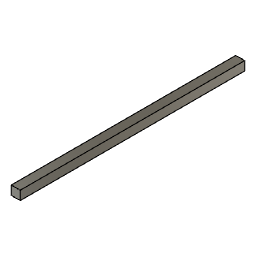
ADR Taskphase build version 1 v1 (Autodesk Fusion 360 archive; units mm, degrees)
design "arms2"
Autodesk Fusion 360 part; units mm, degrees
sketch "Sketch1" plane through (0, 0, 0) normal (0, 1, 0) x (1, 0, 0)
  line L0 (5, -5) -> (-5, -5)
  line L1 (-5, -5) -> (-5, 5)
  line L2 (-5, 5) -> (5, 5)
  line L3 (5, 5) -> (5, -5)
  line L4 (5, -5) -> (-5, 5) construction
  dimension "d1" = 10
  dimension "d2" = 10
  constraint horizontal L0
  constraint perpendicular L0 L1
  constraint parallel L0 L2
  constraint parallel L1 L3
  constraint coincident L4 origin
  measures "d1" distance of L1.end L2.end
  measures "d2" distance of L0.end L1.end
extrude "Extrude1" add sketch "Sketch1" along normal blind 250

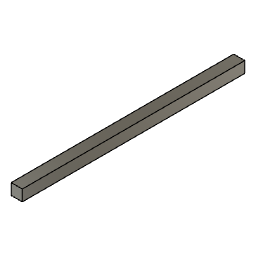
design "gear2"
Autodesk Fusion 360 part; units mm, degrees
sketch "Sketch1" plane through (0, 0, 0) normal (0, 1, 0) x (1, 0, 0)
  line L0 (5, -5) -> (-5, -5)
  line L1 (-5, -5) -> (-5, 5)
  line L2 (-5, 5) -> (5, 5)
  line L3 (5, 5) -> (5, -5)
  line L4 (5, -5) -> (-5, 5) construction
  line L5 (-5, -5) -> (5, 5) construction
  dimension "d1" = 10
  dimension "d2" = 10
  constraint horizontal L0
  constraint perpendicular L0 L1
  constraint parallel L0 L2
  constraint parallel L1 L3
  constraint coincident L4 origin
  constraint coincident L5 origin
  measures "d1" distance of L1.end L2.end
  measures "d2" distance of L0.end L1.end
extrude "Extrude1" add sketch "Sketch1" along normal blind 200

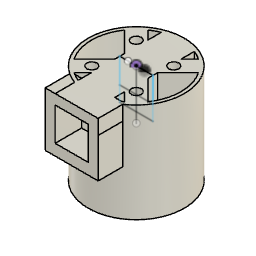
design "motor mount"
Autodesk Fusion 360 part; units mm, degrees
sketch "Sketch1" plane through (0, 0, 0) normal (0, 0, 1) x (1, 0, 0)
  circle A0 centre (0, 0) radius 8
  circle A1 centre (0, 0) radius 9.5
  line L0 (0, 0) -> (5.6569, 5.6569)
  line L1 (0, 0) -> (8, 0) construction
  line L2 (0, 0) -> (5.6569, -5.6569)
  line L3 (0, 0) -> (8.3207, 0) construction
  circle A2 centre (5.6569, 5.6569) radius 1.5
  line L4 (5.6569, -5.6569) -> (6.7175, -6.7175)
  line L5 (5.6569, -5.6569) -> (8.9706, -5.6569) construction
  circle A3 centre (6.7175, -6.7175) radius 1.5
  line L6 (0, 0) -> (-6.7175, 6.7175)
  line L7 (0, 0) -> (10.596, 0) construction
  circle A4 centre (-6.7175, 6.7175) radius 1.5
  line L8 (0, 0) -> (-6.7175, -6.7175)
  line L9 (0, 0) -> (10.7484, 0) construction
  circle A5 centre (-6.7175, -6.7175) radius 1.5
  line L10 (0, 0) -> (1.7678, 1.7678)
  line L11 (0, 0) -> (-1.7678, -1.7678)
  line L12 (-1.7678, -1.7678) -> (-8.2485, 4.713)
  line L13 (-1.7678, -1.7678) -> (7.6131, -11.1486)
  circle A6 centre (0, 0) radius 13.5
  line L14 (-8.2485, 4.713) -> (-11.1486, 7.6131)
  line L15 (1.7678, 1.7678) -> (1.4057, 2.1299)
  line L16 (1.4057, 2.1299) -> (-7.6131, 11.1486)
  line L17 (1.7678, 1.7678) -> (11.1486, -7.6131)
  line L18 (0, 0) -> (-1.7678, 1.7678)
  line L19 (-1.7678, 1.7678) -> (7.6131, 11.1486)
  line L20 (-1.7678, 1.7678) -> (-11.1486, -7.6131)
  line L21 (0, 0) -> (1.7678, -1.7678)
  line L22 (1.7678, -1.7678) -> (11.1486, 7.6131)
  line L23 (1.7678, -1.7678) -> (-7.6131, -11.1486)
  circle A7 centre (0, 0) radius 14.5
  line L24 (0, 0) -> (0, -14.5)
  dimension "d1" = 16
  dimension "d2" = 19
  dimension "d3" = 45
  dimension "d4" = 45
  dimension "d5" = 3
  dimension "d6" = 45
  dimension "d7" = 3
  dimension "d8" = 135
  dimension "d9" = 3
  dimension "d10" = 135
  dimension "d11" = 3
  dimension "d12" = 2.5
  dimension "d13" = 2.5
  dimension "d14" = 27
  dimension "d15" = 2.5
  dimension "d16" = 2.5
  dimension "d17" = 29
  constraint coincident A0.centre A1.centre
  constraint concentric A0 A1
  constraint horizontal L1
  constraint coincident A0 L0.end
  constraint horizontal L3
  constraint coincident A0 L2.end
  constraint coincident L0.end A2.centre
  constraint horizontal L5
  constraint coincident A1 L4.end
  constraint coincident L4.end A3.centre
  constraint horizontal L7
  constraint coincident A1 L6.end
  constraint coincident L6.end A4.centre
  constraint horizontal L9
  constraint coincident A1 L8.end
  constraint coincident L8.end A5.centre
  constraint parallel L0 L10
  constraint perpendicular L6 L11
  constraint coincident A1 L12.end
  constraint perpendicular L8 L12
  constraint perpendicular L11 L13
  constraint concentric A0 A6
  constraint coincident A6 L14.end
  constraint parallel L12 L14
  constraint perpendicular L0 L15
  constraint coincident A6 L16.end
  constraint perpendicular L0 L16
  constraint coincident A6 L17.end
  constraint perpendicular L0 L17
  constraint coincident A6 L13.end
  constraint perpendicular L11 L18
  constraint coincident A6 L19.end
  constraint perpendicular L6 L19
  constraint coincident A6 L20.end
  constraint perpendicular L6 L20
  constraint perpendicular L0 L21
  constraint coincident A6 L22.end
  constraint perpendicular L21 L22
  constraint coincident A6 L23.end
  constraint perpendicular L21 L23
  constraint coincident A7 L24.end
  constraint vertical L24
  measures "d1" diameter of A0
  measures "d2" diameter of A1
  measures "d3" angle of L0 L1
  measures "d4" angle of L2 L3
  measures "d5" diameter of A2
  measures "d6" angle of L4 L5
  measures "d7" diameter of A3
  measures "d8" angle of L6 L7
  measures "d9" diameter of A4
  measures "d10" angle of L8 L9
  measures "d11" diameter of A5
  measures "d12" distance of A0.centre L10.end
  measures "d13" distance of A0.centre L11.end
  measures "d14" diameter of A6
  measures "d15" distance of A0.centre L18.end
  measures "d16" distance of A0.centre L21.end
  measures "d17" diameter of A7
extrude "Extrude1" add sketch "Sketch1" against normal blind 30 contours A0 L0 A2 L17 L22 | A0 A1 A2 L22 | A0 A1 A3 L17 | A0 L2 L17 L22 | L0 L2 L10 L17 L21 L22 | A1 A6 L19 L22 | A0 A1 A3 L13 | A0 L2 L13 L23 | A1 A3 L13 A6 L17 | A0 L0 A2 L15 L16 L19 | L0 L6 L10 L15 L16 L18 L19 | L2 L21 L23 L24 | A0 A1 A2 L19 | L6 L8 L11 L12 L18 L20 | L8 L11 L13 L24 | A0 L8 L13 L23 | A0 L6 L12 L20 | A0 L6 L16 L19 | A0 L8 L12 L20 | A0 A1 A5 L23 | A0 A1 A4 L16 | A1 A4 A6 L14 L16 | A0 A1 A4 L12 | A0 A1 A5 L20 | A1 A5 A6 L20 L23 | A7 makes body 1
sketch "Sketch2" plane through (0, 0, 0) normal (0, 1, 0) x (1, 0, 0)
  line L0 (0, 0) -> (0, 15)
  line L1 (0, 0) -> (2.5, 0)
  line L2 (-2.5, 0) -> (0, 0)
  line L3 (0, 0) -> (5, 0)
  line L4 (5, 0) -> (5, 7.5)
  line L5 (5, 7.5) -> (-5, 7.5)
  line L6 (-5, 7.5) -> (-5, 0)
  line L7 (-5, 0) -> (0, 0)
  line L8 (-5, 0) -> (-5, 12)
  line L9 (-5, 12) -> (5, 12)
  line L10 (5, 12) -> (5, 0)
  dimension "d20" = 2.5
  dimension "d23" = 7.5
  dimension "d24" = 10
  dimension "d33" = 12
  constraint coincident L0.start L1.start
  constraint vertical L0
  constraint perpendicular L0 L1
  constraint perpendicular L0 L2
  constraint perpendicular L0 L3
  constraint perpendicular L3 L4
  constraint perpendicular L0 L5
  constraint perpendicular L3 L6
  constraint perpendicular L6 L7
  constraint perpendicular L7 L8
  constraint perpendicular L0 L9
  constraint perpendicular L3 L10
  measures "d20" distance of L0.start L1.end
  measures "d23" distance of L3.end L4.end
  measures "d24" distance of L4.end L5.end
  measures "d33" distance of L6.end L8.end
extrude "Extrude2" add sketch "Sketch2" against normal blind 19.5 contours L0 L2 L5 L6 L7 L8 | L0 L1 L3 L4 L5 L10 bodies 1
extrude "Extrude3" add sketch "Sketch2" along normal blind 13.5 contours L0 L2 L5 L6 L7 L8 | L0 L1 L3 L4 L5 L10 bodies 1
sketch "Sketch3" plane through (0, -19.5, 0) normal (0, -1, 0) x (1, 0, 0)
  line L0 (5, 0) -> (-5, 0)
  line L1 (-5, 0) -> (-5, -7.5)
  line L2 (-5, -7.5) -> (5, -7.5)
  line L3 (5, -7.5) -> (5, 0)
  line L4 (-5, 0) -> (-5, -0.8052)
  line L5 (0, 0) -> (0, -3)
  line L6 (0, -3) -> (5, -3)
  line L7 (0, -3) -> (-5, -3)
  line L8 (-5, -3) -> (-5, -13)
  line L9 (-5, -13) -> (5, -13)
  line L10 (5, -13) -> (5, -3)
  line L11 (5, -4.437) -> (8, -4.437)
  line L12 (8, -4.437) -> (8, 0)
  line L13 (8, 0) -> (-5, 0)
  line L14 (-5, 0) -> (-8, 0)
  line L15 (-8, 0) -> (-8, -16.3484)
  line L16 (0, -13) -> (0, -13.3484)
  line L17 (0, -13.3484) -> (0, -16.3484)
  line L18 (0, -16.3484) -> (-8, -16.3484)
  line L19 (0, -16.3484) -> (8, -16.3484)
  line L20 (8, -4.437) -> (8, -16.3484)
  dimension "d41" = 3
  dimension "d42" = 5
  dimension "d43" = 10
  dimension "d44" = 3
  dimension "d45" = 3
  dimension "d46" = 3
  constraint coincident L1 L4.end
  constraint coincident L5.start origin
  constraint perpendicular L0 L5
  constraint perpendicular L5 L6
  constraint coincident L1 L7.end
  constraint perpendicular L1 L7
  constraint perpendicular L2 L8
  constraint perpendicular L8 L9
  constraint coincident L10 L11.start
  constraint perpendicular L10 L11
  constraint perpendicular L11 L12
  constraint parallel L0 L13
  constraint coincident L0.end L1.start
  constraint perpendicular L4 L14
  constraint perpendicular L14 L15
  constraint midpoint L9 L16.start
  constraint perpendicular L9 L16
  constraint perpendicular L9 L17
  constraint perpendicular L15 L18
  constraint perpendicular L17 L19
  constraint perpendicular L19 L20
  measures "d41" distance of L5.start L5.end
  measures "d42" distance of L5.end L6.end
  measures "d43" distance of L7.end L8.end
  measures "d44" distance of L11.start L11.end
  measures "d45" distance of L0.end L14.end
  measures "d46" distance of L16.end L17.end
extrude "Extrude6" add sketch "Sketch3" against normal blind 8 bodies 1
extrude "Extrude7" cut sketch "Sketch3" against normal blind 10 contours L1 L2 L3 L6 L7 L8 L10 | L2 L8 L9 L10 bodies 1
extrude "Extrude8" cut 1 faces at (-1.6667, -9.5, -4.5) along direction (0, 1, 0) blind 7 on bodies 1 bodies 1
sketch "Sketch4" plane through (0, 0, -30) normal (0, 0, -1) x (1, 0, 0)
  line L0 (-3.5355, 0) -> (-11.1486, -7.6131)
  arc A0 (-11.1486, 7.6131) -> (-11.1486, -7.6131) centre (0, 0) ccw
  line L1 (-11.1486, 7.6131) -> (-3.5355, 0)
  circle A1 centre (5.6569, -5.6569) radius 1.5
  arc A2 (-7.6131, -11.1486) -> (7.6131, -11.1486) centre (0, 0) ccw
  line L2 (-7.6131, -11.1486) -> (0, -3.5355)
  line L3 (0, -3.5355) -> (7.6131, -11.1486)
  circle A3 centre (-6.7175, 6.7175) radius 1.5
  circle A4 centre (-6.7175, -6.7175) radius 1.5
  line L4 (3.5355, 0) -> (11.1486, 7.6131)
  arc A5 (11.1486, -7.6131) -> (11.1486, 7.6131) centre (0, 0) ccw
  line L5 (11.1486, -7.6131) -> (3.5355, 0)
  circle A6 centre (6.7175, 6.7175) radius 1.5
  arc A7 (7.6131, 11.1486) -> (-7.6131, 11.1486) centre (0, 0) ccw
  line L6 (7.6131, 11.1486) -> (0, 3.5355)
  line L7 (0, 3.5355) -> (-7.6131, 11.1486)
  circle A8 centre (0, 0) radius 14.5
  circle A9 centre (0, 0) radius 13.5
  line L8 (-11.1486, 7.6131) -> (7.6131, -11.1486)
  line L9 (-7.6131, -11.1486) -> (-7.1464, -10.6819)
  line L10 (11.1486, 7.6131) -> (-7.6131, -11.1486)
  line L11 (7.6131, 11.1486) -> (-11.1486, -7.6131)
  line L12 (-7.6131, 11.1486) -> (11.1486, -7.6131)
  dimension "d53" = 27
  constraint concentric A0 A9
  constraint coincident A0.start L1.start
  constraint coincident A2.end L3.end
  constraint coincident A2.start L2.start
  constraint coincident L2 L9.end
  constraint perpendicular L8 L9
  constraint coincident L4.end A5.end
  constraint coincident A7.start L6.start
  constraint coincident L0.end A0.end
  constraint coincident A7.end L7.end
  constraint coincident A5.start L5.start
  measures "d53" diameter of A9
extrude "Extrude9" cut sketch "Sketch4" against normal blind 10 contours L0 L2 A9 L8 L9 L10 L11 | L1 L7 A9 L8 L11 L12 | L3 L5 A9 L8 L10 L12 | L4 L6 A9 L10 L11 L12 bodies 1
extrude "Extrude10" cut 1 faces at (0, -1.1785, -30) along direction (0, 0, 1) blind 10 on bodies 1 bodies 1
sketch "Sketch5" plane through (0, 0, 0) normal (0, 0, 1) x (-1, 0, 0)
  arc A0 (7.6131, 11.1486) -> (7.0711, 11.5) centre (0, 0) ccw
  line L0 (7.6131, 11.1486) -> (5, 8.5355)
  line L1 (5, 8.5355) -> (5, 11.5)
  line L2 (5, 11.5) -> (5, 12.5399)
  arc A1 (7.0711, 11.5) -> (5, 12.5399) centre (0, 0) ccw
  arc A2 (8, 12.0934) -> (5, 13.6107) centre (0, 0) ccw
  line L3 (5, 13.6107) -> (5, 19.5)
  line L4 (5, 19.5) -> (-8, 19.5)
  line L5 (-8, 19.5) -> (-8, 12.0934)
  arc A3 (-8, 12.0934) -> (8, 12.0934) centre (0, 0) ccw
  line L6 (-5, -4.3083) -> (-5, -7.0054)
  arc A4 (-5, -4.3083) -> (-5, -7.0054) centre (-5.6569, -5.6569) ccw
  line L7 (-7.0711, 11.5) -> (-5, 11.5)
  line L8 (-5, 11.5) -> (-5, 8.5355)
  line L9 (-5, 8.5355) -> (-7.6131, 11.1486)
  arc A5 (-7.0711, 11.5) -> (-7.6131, 11.1486) centre (0, 0) ccw
  circle A6 centre (6.7175, 6.7175) radius 1.5
  circle A7 centre (6.7175, -6.7175) radius 1.5
  circle A8 centre (-6.7175, 6.7175) radius 1.5
  line L10 (-5, -1.4645) -> (-11.1486, -7.6131)
  arc A9 (-11.1486, 7.6131) -> (-11.1486, -7.6131) centre (0, 0) ccw
  line L11 (-11.1486, 7.6131) -> (-5, 1.4645)
  line L12 (-5, 1.4645) -> (-5, -1.4645)
  line L13 (5, -12.5399) -> (5, -8.5355)
  line L14 (5, -8.5355) -> (7.6131, -11.1486)
  arc A10 (5, -12.5399) -> (7.6131, -11.1486) centre (0, 0) ccw
  line L15 (5, -1.4645) -> (5, 1.4645)
  line L16 (5, 1.4645) -> (11.1486, 7.6131)
  arc A11 (11.1486, -7.6131) -> (11.1486, 7.6131) centre (0, 0) ccw
  line L17 (11.1486, -7.6131) -> (5, -1.4645)
  arc A12 (-7.6131, -11.1486) -> (-5, -12.5399) centre (0, 0) ccw
  line L18 (-7.6131, -11.1486) -> (-5, -8.5355)
  line L19 (-5, -8.5355) -> (-5, -12.5399)
  line L20 (-5, -1.4645) -> (-3.5355, 0)
  line L21 (-5, 1.4645) -> (-3.5355, 0)
  line L22 (-5, 1.4645) -> (-5, -1.4645)
  line L23 (5, 1.4645) -> (5, -1.4645)
  line L24 (3.5355, 0) -> (3.6807, -0.1451)
  line L25 (3.6807, -0.1451) -> (5, -1.4645)
  line L26 (5, 1.4645) -> (3.5355, 0)
  line L27 (0.0007, -3.5348) -> (3.6081, -7.1423)
  line L28 (3.6081, -7.1423) -> (-3.6067, -7.1423)
  line L29 (-3.6067, -7.1423) -> (0.0007, -3.5348)
  line L30 (0.0007, 3.5298) -> (3.6081, 7.1372)
  line L31 (3.6081, 7.1372) -> (-3.6067, 7.1372)
  line L32 (-3.6067, 7.1372) -> (0.0007, 3.5298)
  circle A13 centre (0, 0) radius 8
  line L33 (3.6807, -0.1451) -> (3.5355, 0)
  dimension "d58" = 16
  constraint coincident L10.start L12.end
  constraint parallel L10 L20
  constraint coincident L11.end L12.start
  constraint perpendicular L20 L21
  constraint coincident L15.end L16.start
  constraint coincident L15.start L17.end
  constraint perpendicular L16 L25
  constraint perpendicular L25 L26
  constraint perpendicular L26 L27
  constraint horizontal L28
  constraint perpendicular L27 L29
  constraint perpendicular L27 L30
  constraint parallel L28 L31
  constraint perpendicular L30 L32
  constraint coincident A0.centre A1.centre
  constraint perpendicular L26 L33
  measures "d58" diameter of A13
copy_body "Body->Comp1" bodies 1 removing the originals makes body 2 in component "motor mount"
sketch "Sketch6" plane through (0, 0, 0) normal (0, 0, 1) x (-1, 0, 0)
  arc A0 (7.6131, 11.1486) -> (7.0711, 11.5) centre (0, 0) ccw
  line L0 (7.6131, 11.1486) -> (5, 8.5355)
  line L1 (5, 8.5355) -> (5, 11.5)
  line L2 (5, 11.5) -> (5, 12.5399)
  arc A1 (7.0711, 11.5) -> (5, 12.5399) centre (0, 0) ccw
  arc A2 (8, 12.0934) -> (5, 13.6107) centre (0, 0) ccw
  line L3 (5, 13.6107) -> (5, 19.5)
  line L4 (5, 19.5) -> (-8, 19.5)
  line L5 (-8, 19.5) -> (-8, 12.0934)
  arc A3 (-8, 12.0934) -> (8, 12.0934) centre (0, 0) ccw
  line L6 (-5, -4.3083) -> (-5, -7.0054)
  arc A4 (-5, -4.3083) -> (-5, -7.0054) centre (-5.6569, -5.6569) ccw
  line L7 (-7.0711, 11.5) -> (-5, 11.5)
  line L8 (-5, 11.5) -> (-5, 8.5355)
  line L9 (-5, 8.5355) -> (-7.6131, 11.1486)
  arc A5 (-7.0711, 11.5) -> (-7.6131, 11.1486) centre (0, 0) ccw
  circle A6 centre (6.7175, 6.7175) radius 1.5
  circle A7 centre (6.7175, -6.7175) radius 1.5
  circle A8 centre (-6.7175, 6.7175) radius 1.5
  line L10 (-5, -1.4645) -> (-11.1486, -7.6131)
  arc A9 (-11.1486, 7.6131) -> (-11.1486, -7.6131) centre (0, 0) ccw
  line L11 (-11.1486, 7.6131) -> (-5, 1.4645)
  line L12 (-5, 1.4645) -> (-5, -1.4645)
  line L13 (5, -12.5399) -> (5, -8.5355)
  line L14 (5, -8.5355) -> (7.6131, -11.1486)
  arc A10 (5, -12.5399) -> (7.6131, -11.1486) centre (0, 0) ccw
  line L15 (5, -1.4645) -> (5, 1.4645)
  line L16 (5, 1.4645) -> (11.1486, 7.6131)
  arc A11 (11.1486, -7.6131) -> (11.1486, 7.6131) centre (0, 0) ccw
  line L17 (11.1486, -7.6131) -> (5, -1.4645)
  arc A12 (-7.6131, -11.1486) -> (-5, -12.5399) centre (0, 0) ccw
  line L18 (-7.6131, -11.1486) -> (-5, -8.5355)
  line L19 (-5, -8.5355) -> (-5, -12.5399)
  circle A13 centre (-5.6569, -5.6569) radius 1.5102
  line L20 (-5, -7.0054) -> (-5, -4.3083)
  constraint concentric A4 A13
  constraint coincident L6.end A4.end
  constraint coincident L6.start A4.start
extrude "Extrude1'" cut sketch "Sketch6" against normal blind 42 contours A13 bodies 2 in component "motor mount"
component "motor mount" placed x (1, 0, 0) y (0, 1, 0) z (0, 0, 1) at (0, 0, 0)

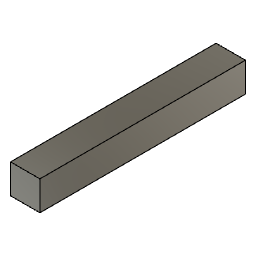
design "landing gear"
Autodesk Fusion 360 part; units mm, degrees
sketch "Sketch1" plane through (0, 0, 0) normal (0, 1, 0) x (1, 0, 0)
  line L0 (5, -5) -> (-5, -5)
  line L1 (-5, -5) -> (-5, 5)
  line L2 (-5, 5) -> (5, 5)
  line L3 (5, 5) -> (5, -5)
  line L4 (5, -5) -> (-5, 5) construction
  line L5 (-5, -5) -> (5, 5) construction
  dimension "d1" = 10
  dimension "d2" = 10
  constraint horizontal L0
  constraint perpendicular L0 L1
  constraint parallel L0 L2
  constraint parallel L1 L3
  constraint coincident L4 origin
  constraint coincident L5 origin
  measures "d1" distance of L1.end L2.end
  measures "d2" distance of L0.end L1.end
extrude "Extrude1" add sketch "Sketch1" along normal blind 70

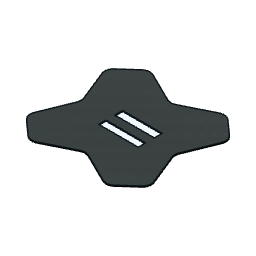
design "baseplate bse medini"
Autodesk Fusion 360 part; units mm, degrees
sketch "Sketch1" plane through (0, 0, 2) normal (0, 0, 1) x (-1, 0, 0)
  line L0 (134.7615, -76.9991) -> (106.995, -8.0888)
  line L1 (39.161, -27.8208) -> (-50, -27.8208)
  line L2 (-50, -27.8208) -> (-50, -10)
  line L3 (-50, -10) -> (39.161, -10)
  line L4 (39.161, -10) -> (39.161, -27.8208)
  line L5 (39.161, 9.6205) -> (-50, 9.6205)
  line L6 (-50, 9.6205) -> (-50, 26.3)
  line L7 (-50, 26.3) -> (39.161, 26.3)
  line L8 (39.161, 26.3) -> (39.161, 9.6205)
  line L9 (-60, -40) -> (-81.5591, -40)
  line L10 (-81.5591, -40) -> (-81.5591, 49.3306)
  line L11 (-81.5591, 49.3306) -> (-60, 49.3306)
  line L12 (-60, 49.3306) -> (-60, -40)
  line L13 (60, -40) -> (81.5591, -40)
  line L14 (60, 49.3306) -> (60, -40)
  line L15 (81.5591, -40) -> (81.5591, 49.3306)
  line L16 (81.5591, 49.3306) -> (60, 49.3306)
  line L17 (129.567, -99.3605) -> (97.0681, -128.5184)
  line L18 (74.8519, -131.5623) -> (8.8599, -98.9538)
  line L19 (-74.8519, -131.5623) -> (-8.8599, -98.9538)
  line L20 (-129.567, -99.3605) -> (-97.0681, -128.5184)
  line L21 (-134.7615, -76.9991) -> (-106.995, -8.0888)
  line L22 (129.567, 98.1323) -> (97.0681, 127.2903)
  line L23 (134.7615, 75.771) -> (106.995, 6.8607)
  line L24 (74.8519, 130.3341) -> (8.8599, 97.7257)
  line L25 (-74.8519, 130.3341) -> (-8.8599, 97.7257)
  line L26 (-134.7615, 75.771) -> (-106.995, 6.8607)
  line L27 (-129.567, 98.1323) -> (-97.0681, 127.2903)
  arc A0 (74.8519, -131.5623) -> (97.0681, -128.5184) centre (83.7118, -113.6318) ccw
  arc A1 (129.567, -99.3605) -> (134.7615, -76.9991) centre (116.2108, -84.4738) ccw
  arc A2 (8.8599, -98.9538) -> (-8.8599, -98.9538) centre (0, -116.8843) ccw
  arc A3 (-97.0681, -128.5184) -> (-74.8519, -131.5623) centre (-83.7118, -113.6318) ccw
  arc A4 (-134.7615, -76.9991) -> (-129.567, -99.3605) centre (-116.2108, -84.4738) ccw
  arc A5 (-129.567, 98.1323) -> (-134.7615, 75.771) centre (-116.2108, 83.2457) ccw
  arc A6 (-74.8519, 130.3341) -> (-97.0681, 127.2903) centre (-83.7118, 112.4036) ccw
  arc A7 (97.0681, 127.2903) -> (74.8519, 130.3341) centre (83.7118, 112.4036) ccw
  arc A8 (134.7615, 75.771) -> (129.567, 98.1323) centre (116.2108, 83.2457) ccw
  arc A9 (106.995, 6.8607) -> (106.995, -8.0888) centre (125.5457, -0.6141) ccw
  arc A10 (-106.995, -8.0888) -> (-106.995, 6.8607) centre (-125.5457, -0.6141) ccw
  arc A11 (-8.8599, 97.7257) -> (8.8599, 97.7257) centre (0, 115.6561) ccw
  arc A12 (8.8599, -98.9538) -> (-8.8599, -98.9538) centre (0, -116.8843) ccw
  arc A13 (50, 26.3) -> (46.3, 30) centre (46.3, 26.3) ccw
  line L28 (50, 26.3) -> (50, -27.8208)
  arc A14 (46.3, -31.5208) -> (50, -27.8208) centre (46.3, -27.8208) ccw
  line L29 (46.3, -31.5208) -> (39.161, -31.5208)
  arc A15 (35.461, -27.8208) -> (39.161, -31.5208) centre (39.161, -27.8208) ccw
  line L30 (35.461, -27.8208) -> (35.461, 26.3)
  arc A16 (39.161, 30) -> (35.461, 26.3) centre (39.161, 26.3) ccw
  line L31 (39.161, 30) -> (46.3, 30)
  arc A17 (24.836, 26.5208) -> (29.836, 31.5208) centre (24.836, 31.5208) ccw
  line L32 (24.836, 26.5208) -> (-25, 26.5208)
  arc A18 (-30, 31.5208) -> (-25, 26.5208) centre (-25, 31.5208) ccw
  line L33 (-30, 31.5208) -> (-30, 35)
  arc A19 (-25, 40) -> (-30, 35) centre (-25, 35) ccw
  line L34 (-25, 40) -> (24.836, 40)
  arc A20 (29.836, 35) -> (24.836, 40) centre (24.836, 35) ccw
  line L35 (29.836, 35) -> (29.836, 31.5208)
  arc A21 (-39.161, -31.5208) -> (-35.461, -27.8208) centre (-39.161, -27.8208) ccw
  line L36 (-39.161, -31.5208) -> (-46.3, -31.5208)
  arc A22 (-50, -27.8208) -> (-46.3, -31.5208) centre (-46.3, -27.8208) ccw
  line L37 (-50, -27.8208) -> (-50, 26.3)
  arc A23 (-46.3, 30) -> (-50, 26.3) centre (-46.3, 26.3) ccw
  line L38 (-46.3, 30) -> (-39.161, 30)
  arc A24 (-35.461, 26.3) -> (-39.161, 30) centre (-39.161, 26.3) ccw
  line L39 (-35.461, 26.3) -> (-35.461, -27.8208)
  line L40 (-30, -35) -> (-30, -31.5208)
  arc A25 (-25, -26.5208) -> (-30, -31.5208) centre (-25, -31.5208) ccw
  line L41 (-25, -26.5208) -> (24.836, -26.5208)
  arc A26 (29.836, -31.5208) -> (24.836, -26.5208) centre (24.836, -31.5208) ccw
  line L42 (29.836, -31.5208) -> (29.836, -35)
  arc A27 (24.836, -40) -> (29.836, -35) centre (24.836, -35) ccw
  line L43 (24.836, -40) -> (-25, -40)
  arc A28 (-30, -35) -> (-25, -40) centre (-25, -35) ccw
  line L44 (3.1623, -61.0541) -> (64.5684, -81.5228)
  arc A29 (64.5684, -81.5228) -> (69.6851, -80.3149) centre (66.1495, -76.7794) ccw
  line L45 (69.6851, -80.3149) -> (90.5258, -59.4742)
  arc A30 (90.5258, -59.4742) -> (91.6327, -54.0817) centre (86.9903, -55.9386) ccw
  line L46 (91.6327, -54.0817) -> (71.4856, -3.7139)
  arc A31 (71.4856, 3.7139) -> (71.4856, -3.7139) centre (80.7703, 0) ccw
  line L47 (71.4856, 3.7139) -> (91.6327, 54.0817)
  arc A32 (91.6327, 54.0817) -> (90.5258, 59.4742) centre (86.9903, 55.9386) ccw
  line L48 (90.5258, 59.4742) -> (69.6851, 80.3149)
  arc A33 (69.6851, 80.3149) -> (64.5684, 81.5228) centre (66.1495, 76.7794) ccw
  line L49 (64.5684, 81.5228) -> (3.1623, 61.0541)
  arc A34 (-3.1623, 61.0541) -> (3.1623, 61.0541) centre (0, 70.5409) ccw
  line L50 (-3.1623, 61.0541) -> (-64.5684, 81.5228)
  arc A35 (-64.5684, 81.5228) -> (-69.6851, 80.3149) centre (-66.1495, 76.7794) ccw
  line L51 (-69.6851, 80.3149) -> (-90.5258, 59.4742)
  arc A36 (-90.5258, 59.4742) -> (-91.6327, 54.0817) centre (-86.9903, 55.9386) ccw
  line L52 (-91.6327, 54.0817) -> (-71.4856, 3.7139)
  arc A37 (-71.4856, -3.7139) -> (-71.4856, 3.7139) centre (-80.7703, 0) ccw
  line L53 (-71.4856, -3.7139) -> (-91.6327, -54.0817)
  arc A38 (-91.6327, -54.0817) -> (-90.5258, -59.4742) centre (-86.9903, -55.9386) ccw
  line L54 (-90.5258, -59.4742) -> (-69.6851, -80.3149)
  arc A39 (-69.6851, -80.3149) -> (-64.5684, -81.5228) centre (-66.1495, -76.7794) ccw
  line L55 (-64.5684, -81.5228) -> (-3.1623, -61.0541)
  arc A40 (3.1623, -61.0541) -> (-3.1623, -61.0541) centre (0, -70.5409) ccw
  dimension "d1" = 20
  dimension "d2" = 20
  dimension "d3" = 20
  dimension "d4" = 20
  constraint horizontal L1
  constraint vertical L2
  constraint horizontal L3
  constraint vertical L4
  constraint horizontal L5
  constraint vertical L6
  constraint horizontal L7
  constraint vertical L8
  constraint horizontal L9
  constraint vertical L10
  constraint horizontal L11
  constraint vertical L12
  constraint tangent L17 A0
  constraint tangent L18 A0
  constraint tangent L0 A1
  constraint tangent L17 A1
  constraint equal A0 A1
  constraint tangent L19 A2
  constraint tangent L18 A2
  constraint equal A0 A2
  constraint tangent L19 A3
  constraint tangent L20 A3
  constraint equal A0 A3
  constraint tangent L20 A4
  constraint tangent L21 A4
  constraint equal A0 A4
  constraint tangent L26 A5
  constraint tangent L27 A5
  constraint equal A0 A5
  constraint tangent L25 A6
  constraint tangent L27 A6
  constraint equal A0 A6
  constraint tangent L22 A7
  constraint tangent L24 A7
  constraint equal A0 A7
  constraint tangent L22 A8
  constraint tangent L23 A8
  constraint equal A0 A8
  constraint tangent L0 A9
  constraint tangent L23 A9
  constraint tangent L21 A10
  constraint tangent L26 A10
  constraint tangent L24 A11
  constraint tangent L25 A11
  constraint coincident L18 A2.start
  constraint coincident L19 A2.end
  constraint tangent L18 A12
  constraint tangent L19 A12
  constraint equal A11 A12
  measures "d1" radius of A0
  measures "d2" radius of A9
  measures "d3" radius of A10
  measures "d4" radius of A11
extrude "Extrude1" add sketch "Sketch1" along normal blind 2 contours L0 L17 L18 L19 L20 L21 L22 L23 L24 L25 L26 L27 A0 A1 A2 A3 A4 A5 A6 A7 A8 A9 A10 A11 A12 | L1 L3 L4 L5 L7 L8 A13 L28 A14 L29 A15 L30 A16 L31 | L1 L40 A25 A26 L42 A27 L43 A28 | L3 L5 L30 L39 | L3 L5 L37 L39 | L1 A21 L36 A22 | L7 A23 L38 A24 | L9 L10 L11 L12 L13 L14 L15 L16 L44 A29 L45 A30 L46 L47 A32 L48 A33 L49 A34 L50 A35 L51 A36 L52 L53 A38 L54 A39 L55 A40 | L9 L10 L11 L12 L52 A37 L53 | L10 L52 A37 L53 | L15 L46 A31 L47 | L13 L14 L15 L16 L46 A31 L47 | A17 L32 A18 L33 A19 L34 A20 L35
sketch "Sketch2" plane through (0, 0, 0) normal (1, 0, 0) x (0, 1, 0)
sketch "Sketch3" plane through (0, 0, 4) normal (0, 0, 1) x (-1, 0, 0)
  line L0 (39.161, -27.8208) -> (-50, -27.8208)
  line L1 (-50, -27.8208) -> (-50, -10)
  line L2 (-50, -10) -> (39.161, -10)
  line L3 (39.161, -10) -> (39.161, -27.8208)
  line L4 (39.161, 26.3) -> (39.161, 9.6205)
  line L5 (39.161, 9.6205) -> (-50, 9.6205)
  line L6 (-50, 9.6205) -> (-50, 26.3)
  line L7 (-50, 26.3) -> (39.161, 26.3)
  arc A0 (74.8519, -131.5623) -> (97.0681, -128.5184) centre (83.7118, -113.6318) ccw
  line L8 (97.0681, -128.5184) -> (129.567, -99.3605)
  arc A1 (129.567, -99.3605) -> (134.7615, -76.9991) centre (116.2108, -84.4738) ccw
  line L9 (134.7615, -76.9991) -> (106.995, -8.0888)
  arc A2 (106.995, 6.8607) -> (106.995, -8.0888) centre (125.5457, -0.6141) ccw
  line L10 (106.995, 6.8607) -> (134.7615, 75.771)
  arc A3 (134.7615, 75.771) -> (129.567, 98.1323) centre (116.2108, 83.2457) ccw
  line L11 (129.567, 98.1323) -> (97.0681, 127.2903)
  arc A4 (97.0681, 127.2903) -> (74.8519, 130.3341) centre (83.7118, 112.4036) ccw
  line L12 (74.8519, 130.3341) -> (8.8599, 97.7257)
  arc A5 (-8.8599, 97.7257) -> (8.8599, 97.7257) centre (0, 115.6561) ccw
  line L13 (-8.8599, 97.7257) -> (-74.8519, 130.3341)
  arc A6 (-74.8519, 130.3341) -> (-97.0681, 127.2903) centre (-83.7118, 112.4036) ccw
  line L14 (-97.0681, 127.2903) -> (-129.567, 98.1323)
  arc A7 (-129.567, 98.1323) -> (-134.7615, 75.771) centre (-116.2108, 83.2457) ccw
  line L15 (-134.7615, 75.771) -> (-106.995, 6.8607)
  arc A8 (-106.995, -8.0888) -> (-106.995, 6.8607) centre (-125.5457, -0.6141) ccw
  line L16 (-106.995, -8.0888) -> (-134.7615, -76.9991)
  arc A9 (-134.7615, -76.9991) -> (-129.567, -99.3605) centre (-116.2108, -84.4738) ccw
  line L17 (-129.567, -99.3605) -> (-97.0681, -128.5184)
  arc A10 (-97.0681, -128.5184) -> (-74.8519, -131.5623) centre (-83.7118, -113.6318) ccw
  line L18 (-74.8519, -131.5623) -> (-8.8599, -98.9538)
  arc A11 (8.8599, -98.9538) -> (-8.8599, -98.9538) centre (0, -116.8843) ccw
  line L19 (8.8599, -98.9538) -> (74.8519, -131.5623)

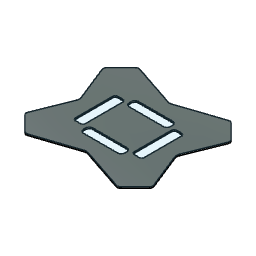
design "baseplate medini"
Autodesk Fusion 360 part; units mm, degrees
sketch "Sketch1" plane through (0, 0, 0) normal (0, 0, 1) x (1, 0, 0)
  line L0 (90, 80) -> (-90, -80) construction
  line L1 (-90, 80) -> (90, -80) construction
  line L2 (-90.5258, 59.4742) -> (-69.6851, 80.3149)
  line L3 (69.6851, 80.3149) -> (90.5258, 59.4742)
  line L4 (-69.6851, -80.3149) -> (-90.5258, -59.4742)
  line L5 (69.6851, -80.3149) -> (90.5258, -59.4742)
  arc A0 (-40, 80) -> (-90, 30) centre (-90, 80) ccw
  arc A1 (90, 30) -> (40, 80) centre (90, 80) ccw
  arc A2 (40, -80) -> (90, -30) centre (90, -80) ccw
  arc A3 (-90, -30) -> (-40, -80) centre (-90, -80) ccw
  line L6 (-24.836, -26.5208) -> (25, -26.5208)
  line L7 (30, -31.5208) -> (30, -35)
  line L8 (25, -40) -> (-24.836, -40)
  line L9 (-29.836, -35) -> (-29.836, -31.5208)
  arc A4 (-24.836, -26.5208) -> (-29.836, -31.5208) centre (-24.836, -31.5208) ccw
  arc A5 (30, -31.5208) -> (25, -26.5208) centre (25, -31.5208) ccw
  arc A6 (25, -40) -> (30, -35) centre (25, -35) ccw
  arc A7 (-29.836, -35) -> (-24.836, -40) centre (-24.836, -35) ccw
  line L10 (-24.836, 26.5208) -> (25, 26.5208)
  line L11 (25, 40) -> (-24.836, 40)
  arc A8 (-24.836, 40) -> (-29.836, 35) centre (-24.836, 35) ccw
  line L12 (-29.836, 35) -> (-29.836, 31.5208)
  arc A9 (-29.836, 31.5208) -> (-24.836, 26.5208) centre (-24.836, 31.5208) ccw
  arc A10 (25, 26.5208) -> (30, 31.5208) centre (25, 31.5208) ccw
  arc A11 (30, 35) -> (25, 40) centre (25, 35) ccw
  line L13 (30, 31.5208) -> (30, 35)
  line L14 (39.161, 31.5208) -> (46.3, 31.5208)
  line L15 (50, 27.8208) -> (50, -26.3)
  line L16 (46.3, -30) -> (39.161, -30)
  line L17 (35.461, -26.3) -> (35.461, 27.8208)
  arc A12 (39.161, 31.5208) -> (35.461, 27.8208) centre (39.161, 27.8208) ccw
  arc A13 (50, 27.8208) -> (46.3, 31.5208) centre (46.3, 27.8208) ccw
  arc A14 (46.3, -30) -> (50, -26.3) centre (46.3, -26.3) ccw
  arc A15 (35.461, -26.3) -> (39.161, -30) centre (39.161, -26.3) ccw
  line L18 (-35.461, -26.3) -> (-35.461, 27.8208)
  line L19 (-50, 27.8208) -> (-50, -26.3)
  line L20 (-39.161, 31.5208) -> (-46.3, 31.5208)
  arc A16 (-35.461, 27.8208) -> (-39.161, 31.5208) centre (-39.161, 27.8208) ccw
  arc A17 (-46.3, 31.5208) -> (-50, 27.8208) centre (-46.3, 27.8208) ccw
  arc A18 (-39.161, -30) -> (-35.461, -26.3) centre (-39.161, -26.3) ccw
  line L21 (-46.3, -30) -> (-39.161, -30)
  arc A19 (-50, -26.3) -> (-46.3, -30) centre (-46.3, -26.3) ccw
  spline S0 degree 5 poles (-36.5447, -32.4841) (-38.2829, -33.9848) (-41.7593, -36.986) (-46.9739, -41.4879) (-53.9268, -47.4905) (-62.6179, -54.9937) (-69.5707, -60.9962) (-74.7854, -65.4981) (-78.2618, -68.4994) (-80, -70) knots 0 0 0 0 0 0 0.2 0.4 0.6 0.8 1 1 1 1 1 1
  line L22 (-91.6327, 54.0817) -> (-71.4856, 3.7139)
  line L23 (-71.4856, -3.7139) -> (-91.6327, -54.0817)
  line L24 (-64.5684, 81.5228) -> (-3.1623, 61.0541)
  line L25 (3.1623, 61.0541) -> (64.5684, 81.5228)
  line L26 (3.1623, -61.0541) -> (64.5684, -81.5228)
  line L27 (-64.5684, -81.5228) -> (-3.1623, -61.0541)
  line L28 (91.6327, 54.0817) -> (71.4856, 3.7139)
  line L29 (71.4856, -3.7139) -> (91.6327, -54.0817)
  arc A20 (-90, 50.9629) -> (-89.6424, 49.106) centre (-85, 50.9629) ccw
  arc A21 (-59.2302, 79.7434) -> (-60.8114, 80) centre (-60.8114, 75) ccw
  arc A22 (-3.1623, 61.0541) -> (3.1623, 61.0541) centre (0, 70.5409) ccw
  arc A23 (60.8114, 80) -> (59.2302, 79.7434) centre (60.8114, 75) ccw
  arc A24 (71.4856, 3.7139) -> (71.4856, -3.7139) centre (80.7703, 0) ccw
  arc A25 (-71.4856, -3.7139) -> (-71.4856, 3.7139) centre (-80.7703, 0) ccw
  arc A26 (-91.6327, -54.0817) -> (-90.5258, -59.4742) centre (-86.9903, -55.9386) ccw
  arc A27 (-69.6851, -80.3149) -> (-64.5684, -81.5228) centre (-66.1495, -76.7794) ccw
  arc A28 (90.5258, -59.4742) -> (91.6327, -54.0817) centre (86.9903, -55.9386) ccw
  arc A29 (64.5684, -81.5228) -> (69.6851, -80.3149) centre (66.1495, -76.7794) ccw
  arc A30 (3.1623, -61.0541) -> (-3.1623, -61.0541) centre (0, -70.5409) ccw
  arc A31 (69.6851, 80.3149) -> (64.5684, 81.5228) centre (66.1495, 76.7794) ccw
  arc A32 (91.6327, 54.0817) -> (90.5258, 59.4742) centre (86.9903, 55.9386) ccw
  arc A33 (91.6327, 54.0817) -> (90.5258, 59.4742) centre (86.9903, 55.9386) ccw
  arc A34 (-90.5258, 59.4742) -> (-91.6327, 54.0817) centre (-86.9903, 55.9386) ccw
  arc A35 (-64.5684, 81.5228) -> (-69.6851, 80.3149) centre (-66.1495, 76.7794) ccw
  dimension "d1" = 180
  dimension "d2" = 160
  dimension "d3" = 100
  dimension "d4" = 100
  dimension "d5" = 5
  dimension "d6" = 5
  dimension "d7" = 3.7
  dimension "d8" = 57.4091
  dimension "d10" = 5
  dimension "d12" = 5
  dimension "d13" = 10
  dimension "d14" = 5
  dimension "d16" = 10
  dimension "d17" = 10
  dimension "d18" = 5
  dimension "d19" = 5
  dimension "d20" = 5
  dimension "d21" = 5
  dimension "d22" = 10
  dimension "d23" = 5
  dimension "d25" = 5
  dimension "d26" = 5
  constraint coincident L0 origin
  constraint coincident L1 origin
  constraint coincident L0.start A1.centre
  constraint coincident L1.start A0.centre
  constraint coincident L0.end A3.centre
  constraint coincident L1.end A2.centre
  constraint perpendicular L2 L3
  constraint perpendicular L4 L5
  constraint horizontal L6
  constraint vertical L7
  constraint horizontal L8
  constraint vertical L9
  constraint tangent L6 A4
  constraint tangent L9 A4
  constraint tangent L6 A5
  constraint tangent L7 A5
  constraint equal A4 A5
  constraint tangent L7 A6
  constraint tangent L8 A6
  constraint equal A4 A6
  constraint tangent L8 A7
  constraint tangent L9 A7
  constraint horizontal L14
  constraint vertical L15
  constraint horizontal L16
  constraint vertical L17
  constraint tangent L14 A12
  constraint tangent L17 A12
  constraint tangent L14 A13
  constraint tangent L15 A13
  constraint equal A12 A13
  constraint tangent L15 A14
  constraint tangent L16 A14
  constraint equal A12 A14
  constraint tangent L16 A15
  constraint tangent L17 A15
  constraint equal A12 A15
  constraint coincident L0 S0.start
  constraint tangent L22 A20
  constraint tangent L24 A21
  constraint tangent L24 A22
  constraint tangent L25 A22
  constraint tangent L25 A23
  constraint tangent L28 A24
  constraint tangent L29 A24
  constraint tangent L22 A25
  constraint tangent L23 A25
  constraint coincident L4 S0.end
  constraint tangent L23 A26
  constraint tangent L4 A26
  constraint tangent L27 A27
  constraint tangent L4 A27
  constraint tangent L29 A28
  constraint tangent L5 A28
  constraint tangent L26 A29
  constraint tangent L5 A29
  constraint tangent L26 A30
  constraint tangent L27 A30
  constraint coincident L25 A23.end
  constraint tangent L3 A31
  constraint tangent L25 A31
  constraint tangent L3 A32
  constraint tangent L28 A32
  constraint coincident L3 A32.end
  constraint coincident L28 A32.start
  constraint tangent L3 A33
  constraint tangent L28 A33
  constraint coincident L22 A20.end
  constraint tangent L22 A34
  constraint tangent L2 A34
  constraint coincident L24 A21.start
  constraint tangent L2 A35
  constraint tangent L24 A35
  measures "d1" distance of L0.end L1.end
  measures "d2" distance of L1.start L0.end
  measures "d3" diameter of A3
  measures "d4" diameter of A2
  measures "d5" radius of A4
  measures "d6" radius of A7
  measures "d7" radius of A12
  measures "d8" distance of S0.start S0.end
  measures "d10" radius of A20
  measures "d12" radius of A21
  measures "d13" radius of A22
  measures "d14" radius of A23
  measures "d16" radius of A24
  measures "d17" radius of A25
  measures "d18" radius of A26
  measures "d19" radius of A27
  measures "d20" radius of A28
  measures "d21" radius of A29
  measures "d22" radius of A30
  measures "d23" radius of A31
  measures "d25" radius of A34
  measures "d26" radius of A35
extrude "Extrude1" add sketch "Sketch1" along normal blind 2
sketch "Sketch2" plane through (0, 0, 2) normal (0, 0, 1) x (-1, 0, 0)
  arc A0 (50, 26.3) -> (46.3, 30) centre (46.3, 26.3) ccw
  line L0 (50, 26.3) -> (50, -27.8208)
  arc A1 (46.3, -31.5208) -> (50, -27.8208) centre (46.3, -27.8208) ccw
  line L1 (46.3, -31.5208) -> (39.161, -31.5208)
  arc A2 (35.461, -27.8208) -> (39.161, -31.5208) centre (39.161, -27.8208) ccw
  line L2 (35.461, -27.8208) -> (35.461, 26.3)
  arc A3 (39.161, 30) -> (35.461, 26.3) centre (39.161, 26.3) ccw
  line L3 (39.161, 30) -> (46.3, 30)
  arc A4 (-39.161, -31.5208) -> (-35.461, -27.8208) centre (-39.161, -27.8208) ccw
  line L4 (-39.161, -31.5208) -> (-46.3, -31.5208)
  arc A5 (-50, -27.8208) -> (-46.3, -31.5208) centre (-46.3, -27.8208) ccw
  line L5 (-50, -27.8208) -> (-50, 26.3)
  arc A6 (-46.3, 30) -> (-50, 26.3) centre (-46.3, 26.3) ccw
  line L6 (-46.3, 30) -> (-39.161, 30)
  arc A7 (-35.461, 26.3) -> (-39.161, 30) centre (-39.161, 26.3) ccw
  line L7 (-35.461, 26.3) -> (-35.461, -27.8208)
  line L8 (-30, -35) -> (-30, -31.5208)
  arc A8 (-25, -26.5208) -> (-30, -31.5208) centre (-25, -31.5208) ccw
  line L9 (-25, -26.5208) -> (24.836, -26.5208)
  arc A9 (29.836, -31.5208) -> (24.836, -26.5208) centre (24.836, -31.5208) ccw
  line L10 (29.836, -31.5208) -> (29.836, -35)
  arc A10 (24.836, -40) -> (29.836, -35) centre (24.836, -35) ccw
  line L11 (24.836, -40) -> (-25, -40)
  arc A11 (-30, -35) -> (-25, -40) centre (-25, -35) ccw
  arc A12 (24.836, 26.5208) -> (29.836, 31.5208) centre (24.836, 31.5208) ccw
  line L12 (24.836, 26.5208) -> (-25, 26.5208)
  arc A13 (-30, 31.5208) -> (-25, 26.5208) centre (-25, 31.5208) ccw
  line L13 (-30, 31.5208) -> (-30, 35)
  arc A14 (-25, 40) -> (-30, 35) centre (-25, 35) ccw
  line L14 (-25, 40) -> (24.836, 40)
  arc A15 (29.836, 35) -> (24.836, 40) centre (24.836, 35) ccw
  line L15 (29.836, 35) -> (29.836, 31.5208)
  line L16 (3.1623, -61.0541) -> (64.5684, -81.5228)
  arc A16 (64.5684, -81.5228) -> (69.6851, -80.3149) centre (66.1495, -76.7794) ccw
  line L17 (69.6851, -80.3149) -> (90.5258, -59.4742)
  arc A17 (90.5258, -59.4742) -> (91.6327, -54.0817) centre (86.9903, -55.9386) ccw
  line L18 (91.6327, -54.0817) -> (71.4856, -3.7139)
  arc A18 (71.4856, 3.7139) -> (71.4856, -3.7139) centre (80.7703, 0) ccw
  line L19 (71.4856, 3.7139) -> (91.6327, 54.0817)
  arc A19 (91.6327, 54.0817) -> (90.5258, 59.4742) centre (86.9903, 55.9386) ccw
  line L20 (90.5258, 59.4742) -> (69.6851, 80.3149)
  arc A20 (69.6851, 80.3149) -> (64.5684, 81.5228) centre (66.1495, 76.7794) ccw
  line L21 (64.5684, 81.5228) -> (3.1623, 61.0541)
  arc A21 (-3.1623, 61.0541) -> (3.1623, 61.0541) centre (0, 70.5409) ccw
  line L22 (-3.1623, 61.0541) -> (-64.5684, 81.5228)
  arc A22 (-64.5684, 81.5228) -> (-69.6851, 80.3149) centre (-66.1495, 76.7794) ccw
  line L23 (-69.6851, 80.3149) -> (-90.5258, 59.4742)
  arc A23 (-90.5258, 59.4742) -> (-91.6327, 54.0817) centre (-86.9903, 55.9386) ccw
  line L24 (-91.6327, 54.0817) -> (-71.4856, 3.7139)
  arc A24 (-71.4856, -3.7139) -> (-71.4856, 3.7139) centre (-80.7703, 0) ccw
  line L25 (-71.4856, -3.7139) -> (-91.6327, -54.0817)
  arc A25 (-91.6327, -54.0817) -> (-90.5258, -59.4742) centre (-86.9903, -55.9386) ccw
  line L26 (-90.5258, -59.4742) -> (-69.6851, -80.3149)
  arc A26 (-69.6851, -80.3149) -> (-64.5684, -81.5228) centre (-66.1495, -76.7794) ccw
  line L27 (-64.5684, -81.5228) -> (-3.1623, -61.0541)
  arc A27 (3.1623, -61.0541) -> (-3.1623, -61.0541) centre (0, -70.5409) ccw
sketch "Sketch3" plane through (0, 0, 2) normal (0, 0, 1) x (-1, 0, 0)
  arc A0 (50, 26.3) -> (46.3, 30) centre (46.3, 26.3) ccw
  line L0 (50, 26.3) -> (50, -27.8208)
  arc A1 (46.3, -31.5208) -> (50, -27.8208) centre (46.3, -27.8208) ccw
  line L1 (46.3, -31.5208) -> (39.161, -31.5208)
  arc A2 (35.461, -27.8208) -> (39.161, -31.5208) centre (39.161, -27.8208) ccw
  line L2 (35.461, -27.8208) -> (35.461, 26.3)
  arc A3 (39.161, 30) -> (35.461, 26.3) centre (39.161, 26.3) ccw
  line L3 (39.161, 30) -> (46.3, 30)
  arc A4 (-39.161, -31.5208) -> (-35.461, -27.8208) centre (-39.161, -27.8208) ccw
  line L4 (-39.161, -31.5208) -> (-46.3, -31.5208)
  arc A5 (-50, -27.8208) -> (-46.3, -31.5208) centre (-46.3, -27.8208) ccw
  line L5 (-50, -27.8208) -> (-50, 26.3)
  arc A6 (-46.3, 30) -> (-50, 26.3) centre (-46.3, 26.3) ccw
  line L6 (-46.3, 30) -> (-39.161, 30)
  arc A7 (-35.461, 26.3) -> (-39.161, 30) centre (-39.161, 26.3) ccw
  line L7 (-35.461, 26.3) -> (-35.461, -27.8208)
  line L8 (-30, -35) -> (-30, -31.5208)
  arc A8 (-25, -26.5208) -> (-30, -31.5208) centre (-25, -31.5208) ccw
  line L9 (-25, -26.5208) -> (24.836, -26.5208)
  arc A9 (29.836, -31.5208) -> (24.836, -26.5208) centre (24.836, -31.5208) ccw
  line L10 (29.836, -31.5208) -> (29.836, -35)
  arc A10 (24.836, -40) -> (29.836, -35) centre (24.836, -35) ccw
  line L11 (24.836, -40) -> (-25, -40)
  arc A11 (-30, -35) -> (-25, -40) centre (-25, -35) ccw
  arc A12 (24.836, 26.5208) -> (29.836, 31.5208) centre (24.836, 31.5208) ccw
  line L12 (24.836, 26.5208) -> (-25, 26.5208)
  arc A13 (-30, 31.5208) -> (-25, 26.5208) centre (-25, 31.5208) ccw
  line L13 (-30, 31.5208) -> (-30, 35)
  arc A14 (-25, 40) -> (-30, 35) centre (-25, 35) ccw
  line L14 (-25, 40) -> (24.836, 40)
  arc A15 (29.836, 35) -> (24.836, 40) centre (24.836, 35) ccw
  line L15 (29.836, 35) -> (29.836, 31.5208)
  line L16 (3.1623, -61.0541) -> (64.5684, -81.5228)
  arc A16 (64.5684, -81.5228) -> (69.6851, -80.3149) centre (66.1495, -76.7794) ccw
  line L17 (69.6851, -80.3149) -> (90.5258, -59.4742)
  arc A17 (90.5258, -59.4742) -> (91.6327, -54.0817) centre (86.9903, -55.9386) ccw
  line L18 (91.6327, -54.0817) -> (71.4856, -3.7139)
  arc A18 (71.4856, 3.7139) -> (71.4856, -3.7139) centre (80.7703, 0) ccw
  line L19 (71.4856, 3.7139) -> (91.6327, 54.0817)
  arc A19 (91.6327, 54.0817) -> (90.5258, 59.4742) centre (86.9903, 55.9386) ccw
  line L20 (90.5258, 59.4742) -> (69.6851, 80.3149)
  arc A20 (69.6851, 80.3149) -> (64.5684, 81.5228) centre (66.1495, 76.7794) ccw
  line L21 (64.5684, 81.5228) -> (3.1623, 61.0541)
  arc A21 (-3.1623, 61.0541) -> (3.1623, 61.0541) centre (0, 70.5409) ccw
  line L22 (-3.1623, 61.0541) -> (-64.5684, 81.5228)
  arc A22 (-64.5684, 81.5228) -> (-69.6851, 80.3149) centre (-66.1495, 76.7794) ccw
  line L23 (-69.6851, 80.3149) -> (-90.5258, 59.4742)
  arc A23 (-90.5258, 59.4742) -> (-91.6327, 54.0817) centre (-86.9903, 55.9386) ccw
  line L24 (-91.6327, 54.0817) -> (-71.4856, 3.7139)
  arc A24 (-71.4856, -3.7139) -> (-71.4856, 3.7139) centre (-80.7703, 0) ccw
  line L25 (-71.4856, -3.7139) -> (-91.6327, -54.0817)
  arc A25 (-91.6327, -54.0817) -> (-90.5258, -59.4742) centre (-86.9903, -55.9386) ccw
  line L26 (-90.5258, -59.4742) -> (-69.6851, -80.3149)
  arc A26 (-69.6851, -80.3149) -> (-64.5684, -81.5228) centre (-66.1495, -76.7794) ccw
  line L27 (-64.5684, -81.5228) -> (-3.1623, -61.0541)
  arc A27 (3.1623, -61.0541) -> (-3.1623, -61.0541) centre (0, -70.5409) ccw
sketch "Sketch4" plane through (0, 0, 2) normal (0, 0, 1) x (-1, 0, 0)
  arc A0 (50, 26.3) -> (46.3, 30) centre (46.3, 26.3) ccw
  line L0 (50, 26.3) -> (50, -27.8208)
  arc A1 (46.3, -31.5208) -> (50, -27.8208) centre (46.3, -27.8208) ccw
  line L1 (46.3, -31.5208) -> (39.161, -31.5208)
  arc A2 (35.461, -27.8208) -> (39.161, -31.5208) centre (39.161, -27.8208) ccw
  line L2 (35.461, -27.8208) -> (35.461, 26.3)
  arc A3 (39.161, 30) -> (35.461, 26.3) centre (39.161, 26.3) ccw
  line L3 (39.161, 30) -> (46.3, 30)
  arc A4 (-39.161, -31.5208) -> (-35.461, -27.8208) centre (-39.161, -27.8208) ccw
  line L4 (-39.161, -31.5208) -> (-46.3, -31.5208)
  arc A5 (-50, -27.8208) -> (-46.3, -31.5208) centre (-46.3, -27.8208) ccw
  line L5 (-50, -27.8208) -> (-50, 26.3)
  arc A6 (-46.3, 30) -> (-50, 26.3) centre (-46.3, 26.3) ccw
  line L6 (-46.3, 30) -> (-39.161, 30)
  arc A7 (-35.461, 26.3) -> (-39.161, 30) centre (-39.161, 26.3) ccw
  line L7 (-35.461, 26.3) -> (-35.461, -27.8208)
  line L8 (-30, -35) -> (-30, -31.5208)
  arc A8 (-25, -26.5208) -> (-30, -31.5208) centre (-25, -31.5208) ccw
  line L9 (-25, -26.5208) -> (24.836, -26.5208)
  arc A9 (29.836, -31.5208) -> (24.836, -26.5208) centre (24.836, -31.5208) ccw
  line L10 (29.836, -31.5208) -> (29.836, -35)
  arc A10 (24.836, -40) -> (29.836, -35) centre (24.836, -35) ccw
  line L11 (24.836, -40) -> (-25, -40)
  arc A11 (-30, -35) -> (-25, -40) centre (-25, -35) ccw
  arc A12 (24.836, 26.5208) -> (29.836, 31.5208) centre (24.836, 31.5208) ccw
  line L12 (24.836, 26.5208) -> (-25, 26.5208)
  arc A13 (-30, 31.5208) -> (-25, 26.5208) centre (-25, 31.5208) ccw
  line L13 (-30, 31.5208) -> (-30, 35)
  arc A14 (-25, 40) -> (-30, 35) centre (-25, 35) ccw
  line L14 (-25, 40) -> (24.836, 40)
  arc A15 (29.836, 35) -> (24.836, 40) centre (24.836, 35) ccw
  line L15 (29.836, 35) -> (29.836, 31.5208)
  line L16 (3.1623, -61.0541) -> (64.5684, -81.5228)
  arc A16 (64.5684, -81.5228) -> (69.6851, -80.3149) centre (66.1495, -76.7794) ccw
  line L17 (69.6851, -80.3149) -> (90.5258, -59.4742)
  arc A17 (90.5258, -59.4742) -> (91.6327, -54.0817) centre (86.9903, -55.9386) ccw
  line L18 (91.6327, -54.0817) -> (71.4856, -3.7139)
  arc A18 (71.4856, 3.7139) -> (71.4856, -3.7139) centre (80.7703, 0) ccw
  line L19 (71.4856, 3.7139) -> (91.6327, 54.0817)
  arc A19 (91.6327, 54.0817) -> (90.5258, 59.4742) centre (86.9903, 55.9386) ccw
  line L20 (90.5258, 59.4742) -> (69.6851, 80.3149)
  arc A20 (69.6851, 80.3149) -> (64.5684, 81.5228) centre (66.1495, 76.7794) ccw
  line L21 (64.5684, 81.5228) -> (3.1623, 61.0541)
  arc A21 (-3.1623, 61.0541) -> (3.1623, 61.0541) centre (0, 70.5409) ccw
  line L22 (-3.1623, 61.0541) -> (-64.5684, 81.5228)
  arc A22 (-64.5684, 81.5228) -> (-69.6851, 80.3149) centre (-66.1495, 76.7794) ccw
  line L23 (-69.6851, 80.3149) -> (-90.5258, 59.4742)
  arc A23 (-90.5258, 59.4742) -> (-91.6327, 54.0817) centre (-86.9903, 55.9386) ccw
  line L24 (-91.6327, 54.0817) -> (-71.4856, 3.7139)
  arc A24 (-71.4856, -3.7139) -> (-71.4856, 3.7139) centre (-80.7703, 0) ccw
  line L25 (-71.4856, -3.7139) -> (-91.6327, -54.0817)
  arc A25 (-91.6327, -54.0817) -> (-90.5258, -59.4742) centre (-86.9903, -55.9386) ccw
  line L26 (-90.5258, -59.4742) -> (-69.6851, -80.3149)
  arc A26 (-69.6851, -80.3149) -> (-64.5684, -81.5228) centre (-66.1495, -76.7794) ccw
  line L27 (-64.5684, -81.5228) -> (-3.1623, -61.0541)
  arc A27 (3.1623, -61.0541) -> (-3.1623, -61.0541) centre (0, -70.5409) ccw
